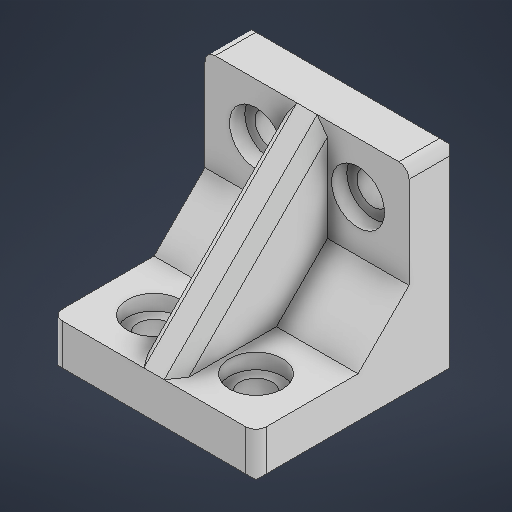
# Autodesk Inventor part: T
Saved by Autodesk Inventor 2026.2 (Build 302298010, 298A)
## iProperties
Created: 2026-04-16
Part Number: T
Material: Genérico
Document SubType Name: Modeling
Designer: Jose Carlos
Density: 1 g/cm^3
Appearance: Valor por defecto
Author: Jose Carlos
Autodesk Inventor part; units mm, degrees
ref_plane "YZ Plane" through (0, 0, 0) normal (1, 0, 0) x (0, 1, 0)
ref_plane "XZ Plane" through (0, 0, 0) normal (0, 1, 0) x (-1, 0, 0)
ref_plane "XY Plane" through (0, 0, 0) normal (0, 0, 1) x (1, 0, 0)
sketch "Boceto1" plane through (0, 0, 0) normal (0, 0, 1) x (1, 0, 0)
  line L0 (10, 0) -> (-10, 0)
  line L1 (-10, 0) -> (-10, 20)
  line L2 (-10, 20) -> (10, 20)
  line L3 (10, 20) -> (10, 0)
  point P0 (0, 0)
  point P1 (0, 0)
  dimension "d0" = 20
  dimension "d1" = 20
  constraints: 8 end point, 2 parallel, 1 coincident, 1 horizontal, 1 midpoint, 1 perpendicular
  measures "d0" distance of L0.end L1.end
  measures "d1" distance of L1.end L2.end
extrude "Extrusión1" add sketch "Boceto1" along normal blind 5
sketch "Boceto2" plane through (0, 0, 0) normal (0, 0, 1) x (1, 0, 0)
  line L0 (-10, 0) -> (10, 0) construction
  line L1 (-10, 0) -> (10, 0)
  line L2 (10, 0) -> (10, 5)
  line L3 (10, 5) -> (-10, 5)
  line L4 (-10, 5) -> (-10, 0)
  point P0 (0, 0)
  dimension "d4" = 5
  constraints: 8 end point, 2 parallel, 1 horizontal, 1 perpendicular
  measures "d4" distance of L3.end L0.start
extrude "Extrusión2" add sketch "Boceto2" along normal blind 20
sketch "Boceto3" plane through (0, 0, 5) normal (0, 0, 1) x (1, 0, 0)
  line L0 (-10, 20) -> (-10, 5) construction
  line L1 (10, 20) -> (-10, 20) construction
  line L2 (10, 5) -> (10, 20) construction
  point P0 (0, 0)
  point P1 (-5, 15)
  point P2 (5, 15)
  dimension "d7" = 5
  dimension "d8" = 5
  dimension "d9" = 5
  dimension "d10" = 5
  measures "d7" distance from line of L0 point (-5, 15)
  measures "d8" distance from line of L1 point (-5, 15)
  measures "d9" distance from line of L2 point (5, 15)
  measures "d10" distance from line of L1 point (5, 15)
sketch "Boceto4" plane through (-10, 5, 5) normal (0, 1, 0) x (1, 0, 0)
  line L0 (0, 0) -> (0, -15) construction
  line L1 (20, -15) -> (0, -15) construction
  line L2 (20, 0) -> (20, -15) construction
  point P0 (10, 5)
  point P1 (5, -10)
  point P2 (15, -10)
  dimension "d14" = 5
  dimension "d15" = 5
  dimension "d16" = 5
  dimension "d17" = 5
  measures "d14" distance from line of L0 point (5, -10)
  measures "d15" distance from line of L1 point (5, -10)
  measures "d16" distance from line of L1 point (15, -10)
  measures "d17" distance from line of L2 point (15, -10)
hole "Agujero1" at (-5, 5, 15) at (5, 5, 15) direction (0, -1, 0) diameter 3.2 end through all counterbore diameter 5.2 counterbore depth 1.5
hole "Agujero2" at (-5, 15, 5) at (5, 15, 5) direction (0, 0, -1) diameter 3.2 end through all counterbore diameter 5.2 counterbore depth 1.5
sketch "Boceto5" plane through (0, 0, 0) normal (1, 0, 0) x (0, 1, 0)
  line L0 (5, 5) -> (5, 20) construction
  line L1 (5, 20) -> (20, 5)
  line L2 (20, 5) -> (5, 5) construction
  line L3 (5, 5) -> (20, 5) construction
  line L4 (5, 20) -> (5, 5)
  line L5 (20, 5) -> (5, 5)
  point P0 (0, 0)
  dimension "d32" = 45
  dimension "d33" = 15
  constraints: 6 end point, 2 collinear, 2 point on line
  measures "d32" angle of L2 L1
  measures "d33" distance from line of L3 L1.start
extrude "Extrusión4" add sketch "Boceto5" along normal mid plane 4
sketch "Boceto6" plane through (0, 0, 0) normal (1, 0, 0) x (0, 1, 0)
  line L0 (5, 5) -> (5, 20) construction
  line L1 (5, 10) -> (10, 5)
  line L2 (5, 5) -> (20, 5) construction
  line L3 (5, 5) -> (10, 5)
  line L4 (5, 10) -> (5, 5)
  point P0 (0, 0)
  dimension "d36" = 45
  dimension "d37" = 5
  constraints: 6 end point, 2 point on line, 1 collinear, 1 perpendicular
  measures "d36" angle of L2 L1
  measures "d37" distance of L0.start L1.start
extrude "Extrusión5" add sketch "Boceto6" along normal mid plane 20
chamfer "Chaflán1" distance 1 angle 45 9 edges at (-10, 0, 10) (0, 0, 20) (10, 0, 10) (0, 0, 0) (-10, 10, 0) (10, 10, 0) (0, 20, 0) (-2, 12.5, 12.5) (2, 12.5, 12.5)
fillet "Empalme1" radius 1 4 edges at (-10, 3, 20) (-10, 20, 3) (10, 20, 3) (10, 3, 20)
